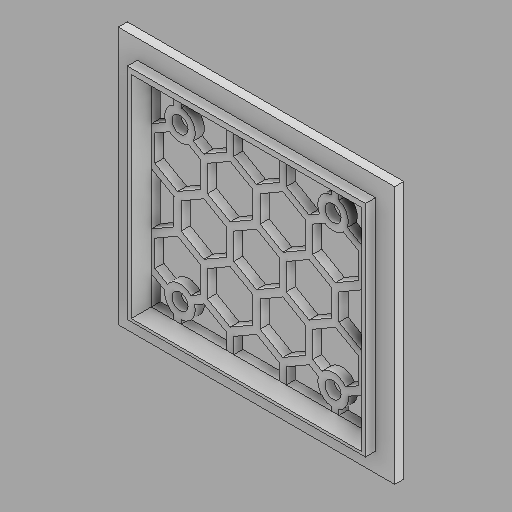
# Autodesk Inventor part: First_Stage_HexGrill
Saved by Autodesk Inventor 2025.2 (Build 292293000, 293)
## iProperties
Created: 2024-12-06
Part Number: First_Stage_HexGrill
Material: Generic
Document SubType Name: Modeling
Designer: Paul Linke
Density: 1 g/cm^3
Appearance: Default
Author: Paul Linke
Autodesk Inventor part; units mm, degrees
ref_plane "YZ Plane" through (0, 0, 0) normal (1, 0, 0) x (0, 1, 0)
ref_plane "XZ Plane" through (0, 0, 0) normal (0, 1, 0) x (-1, 0, 0)
ref_plane "Work Plane1" through (0, 0, 0) normal (0, 0, 1) x (1, 0, 0)
sketch "Sketch1" plane through (0, 0, 0) normal (0, 0, 1) x (1, 0, 0)
  line L0 (-29, 27) -> (-29, -27) projected
  line L1 (-25, -27) -> (-29, -27) projected
  line L2 (-25, 23) -> (-25, -27) projected
  line L3 (25, 23) -> (-25, 23) projected
  line L4 (25, -27) -> (25, 23) projected
  line L5 (29, -27) -> (25, -27) projected
  line L6 (29, -27) -> (29, 27) projected
  line L7 (-29, 27) -> (29, 27) projected
  line L8 (-29, 27) -> (-29, -27) projected
  line L9 (-25, -27) -> (-29, -27) projected
  line L10 (-25, 23) -> (-25, -27) projected
  line L11 (25, 23) -> (-25, 23) projected
  line L12 (25, -27) -> (25, 23) projected
  line L13 (29, -27) -> (25, -27) projected
  line L14 (29, -27) -> (29, 27) projected
  line L15 (-29, 27) -> (29, 27) projected
  line L16 (29, -27) -> (-29, -27)
  line L17 (-29, -27) -> (-29, 27)
  line L18 (-29, 27) -> (29, 27)
  line L19 (29, 27) -> (29, -27)
  line L20 (28.9, -27) -> (-28.9, -27)
  line L21 (-28.9, -27) -> (-28.9, 26.9)
  line L22 (-28.9, 26.9) -> (28.9, 26.9)
  line L23 (28.9, 26.9) -> (28.9, -27)
  line L24 (25, -27) -> (-25, -27)
  line L25 (-25, -27) -> (-25, 23)
  line L26 (-25, 23) -> (25, 23)
  line L27 (25, 23) -> (25, -23)
  line L28 (66.972, -23) -> (25, -23) projected
  line L29 (-25, -23) -> (-107.0316, -23) projected
  line L30 (-25, -23) -> (-25, -26.9)
  dimension "d0" = 0.1
  dimension "d1" = 0.1
  dimension "d2" = 0.1
  constraints: 26 end point, 6 parallel, 3 horizontal, 3 perpendicular, 2 point on line
  measures "d0" distance between parallel lines of L6 L23
  measures "d1" distance between parallel lines of L0 L21
  measures "d2" distance between parallel lines of L18 L22
extrude "Extrusion1" add sketch "Sketch1" along normal blind 1.9 contours L29 L2 L1 L21 | L21 L22 L23 L28 L4 L3 L2 L29 | L2 L3 L4 L16 | L23 L5 L4 L28
sketch "Sketch3" plane through (0, 0, 1.9) normal (0, 0, 1) x (1, 0, 0)
  line L0 (66.972, -23) -> (25, -23) projected
  line L1 (-25, -23) -> (-107.0316, -23) projected
  line L2 (25, 23) -> (25, -23) projected
  line L3 (-25, 23) -> (25, 23) projected
  line L4 (-25, -23) -> (-25, 23) projected
  line L5 (24.9, -23) -> (-24.9, -23)
  line L6 (-24.9, -23) -> (-24.9, 22.9)
  line L7 (-24.9, 22.9) -> (24.9, 22.9)
  line L8 (24.9, 22.9) -> (24.9, -23)
  point P0 (0, 0)
  dimension "d18" = 0.1
  dimension "d19" = 0.1
  dimension "d20" = 0.1
  constraints: 8 end point, 2 parallel, 1 collinear, 1 horizontal, 1 perpendicular
  measures "d18" distance between parallel lines of L2 L8
  measures "d19" distance between parallel lines of L3 L7
  measures "d20" distance between parallel lines of L4 L6
extrude "Extrusion3" add sketch "Sketch3" along normal blind 2.1
sketch "Sketch4" plane through (0, 0, 4) normal (0, 0, 1) x (1, 0, 0)
  line L0 (-24.9, -23) -> (24.9, -23) projected
  line L1 (24.9, 22.9) -> (-24.9, 22.9) projected
  line L2 (-24.9, 22.9) -> (-24.9, -23) projected
  line L3 (-24.9, -23) -> (24.9, -23) projected
  line L4 (24.9, -23) -> (24.9, 22.9) projected
  line L5 (24.9, -23) -> (-24.9, 22.9) construction
  line L6 (24.9, 22.9) -> (-24.9, -23) construction
  line L7 (22, -20.3271) -> (-22, -20.3271)
  line L8 (-22, -20.3271) -> (-22, 19.6729)
  line L9 (-22, 19.6729) -> (22, 19.6729)
  line L10 (22, 19.6729) -> (22, -20.3271)
  point P0 (0, 0)
  dimension "d23" = 44
  dimension "d24" = 40
  constraints: 12 end point, 2 parallel, 2 point on line, 1 horizontal, 1 perpendicular
  measures "d23" distance between parallel lines of L8 L10
  measures "d24" distance between parallel lines of L9 L7
extrude "Extrusion4" cut sketch "Sketch4" against normal blind 2.1 contours L7 L8 L9 L10
chamfer "Chamfer1" distance 2.1 angle 45 4 edges at (0, -20.3271, 4) (-22, -0.3271, 4) (0, 19.6729, 4) (22, -0.3271, 4)
sketch "Sketch5" plane through (0, 0, 1.9) normal (0, 0, 1) x (1, 0, 0)
  line L0 (-43.092, -0.7164) -> (45.2522, -0.7164) construction
  line L1 (-44, 4.7684) -> (-39.25, 2.026)
  line L2 (-39.25, 2.026) -> (-39.25, -3.4588)
  line L3 (-39.25, -3.4588) -> (-44, -6.2012)
  line L4 (-44, -6.2012) -> (-48.75, -3.4588)
  line L5 (-48.75, -3.4588) -> (-48.75, 2.026)
  line L6 (-48.75, 2.026) -> (-44, 4.7684)
  line L7 (-44, 4.7684) -> (-44, -6.2012) construction
  circle A0 centre (-16, 15.6729) radius 1.7
  circle A1 centre (16, 15.6729) radius 1.7
  circle A2 centre (-16, -16.3271) radius 1.7
  circle A3 centre (16, -16.3271) radius 1.7
  line L8 (-24.1, -22.4271) -> (-22, -20.3271) projected
  line L9 (-16, 15.6729) -> (-22, 15.6729) construction
  line L10 (-22, -20.3271) -> (-22, 19.6729) projected
  line L11 (16, 15.6729) -> (22, 15.6729) construction
  line L12 (22, 19.6729) -> (22, -20.3271) projected
  line L13 (-16, 15.6729) -> (-16, 19.6729) construction
  line L14 (-22, 19.6729) -> (22, 19.6729) projected
  line L15 (-16, -16.3271) -> (-16, -20.3271) construction
  line L16 (22, -20.3271) -> (-22, -20.3271) construction
  line L17 (-44, -0.7164) -> (-41.625, 3.3972) construction
  line L18 (-28.25, 2.026) -> (-28.25, -3.4588)
  line L19 (-28.25, -3.4588) -> (-33, -6.2012)
  line L20 (-33, 4.7684) -> (-28.25, 2.026)
  line L21 (-33, -6.2012) -> (-37.75, -3.4588)
  line L22 (-37.75, -3.4588) -> (-37.75, 2.026)
  line L23 (-37.75, 2.026) -> (-33, 4.7684)
  line L24 (-17.25, 2.026) -> (-17.25, -3.4588)
  line L25 (-17.25, -3.4588) -> (-22, -6.2012)
  line L26 (-22, 4.7684) -> (-17.25, 2.026)
  line L27 (-22, -6.2012) -> (-26.75, -3.4588)
  line L28 (-26.75, -3.4588) -> (-26.75, 2.026)
  line L29 (-26.75, 2.026) -> (-22, 4.7684)
  line L30 (-6.25, 2.026) -> (-6.25, -3.4588)
  line L31 (-6.25, -3.4588) -> (-11, -6.2012)
  line L32 (-11, 4.7684) -> (-6.25, 2.026)
  line L33 (-11, -6.2012) -> (-15.75, -3.4588)
  line L34 (-15.75, -3.4588) -> (-15.75, 2.026)
  line L35 (-15.75, 2.026) -> (-11, 4.7684)
  line L36 (4.75, 2.026) -> (4.75, -3.4588)
  line L37 (4.75, -3.4588) -> (0, -6.2012)
  line L38 (0, 4.7684) -> (4.75, 2.026)
  line L39 (0, -6.2012) -> (-4.75, -3.4588)
  line L40 (-4.75, -3.4588) -> (-4.75, 2.026)
  line L41 (-4.75, 2.026) -> (0, 4.7684)
  line L42 (15.75, 2.026) -> (15.75, -3.4588)
  line L43 (15.75, -3.4588) -> (11, -6.2012)
  line L44 (11, 4.7684) -> (15.75, 2.026)
  line L45 (11, -6.2012) -> (6.25, -3.4588)
  line L46 (6.25, -3.4588) -> (6.25, 2.026)
  line L47 (6.25, 2.026) -> (11, 4.7684)
  line L48 (26.75, 2.026) -> (26.75, -3.4588)
  line L49 (26.75, -3.4588) -> (22, -6.2012)
  line L50 (22, 4.7684) -> (26.75, 2.026)
  line L51 (22, -6.2012) -> (17.25, -3.4588)
  line L52 (17.25, -3.4588) -> (17.25, 2.026)
  line L53 (17.25, 2.026) -> (22, 4.7684)
  line L54 (37.75, 2.026) -> (37.75, -3.4588)
  line L55 (37.75, -3.4588) -> (33, -6.2012)
  line L56 (33, 4.7684) -> (37.75, 2.026)
  line L57 (33, -6.2012) -> (28.25, -3.4588)
  line L58 (28.25, -3.4588) -> (28.25, 2.026)
  line L59 (28.25, 2.026) -> (33, 4.7684)
  line L60 (48.75, 2.026) -> (48.75, -3.4588)
  line L61 (48.75, -3.4588) -> (44, -6.2012)
  line L62 (44, 4.7684) -> (48.75, 2.026)
  line L63 (44, -6.2012) -> (39.25, -3.4588)
  line L64 (39.25, -3.4588) -> (39.25, 2.026)
  line L65 (39.25, 2.026) -> (44, 4.7684)
  line L66 (59.75, 2.026) -> (59.75, -3.4588)
  line L67 (59.75, -3.4588) -> (55, -6.2012)
  line L68 (55, 4.7684) -> (59.75, 2.026)
  line L69 (55, -6.2012) -> (50.25, -3.4588)
  line L70 (50.25, -3.4588) -> (50.25, 2.026)
  line L71 (50.25, 2.026) -> (55, 4.7684)
  line L72 (-11.75, 6.0675) -> (-16.5, 3.3251)
  line L73 (-11.75, 11.5523) -> (-11.75, 6.0675)
  line L74 (-16.5, 14.2947) -> (-11.75, 11.5523)
  line L75 (-5.5, 3.3251) -> (-10.25, 6.0675)
  line L76 (-10.25, 11.5523) -> (-5.5, 14.2947)
  line L77 (-0.75, 6.0675) -> (-5.5, 3.3251)
  line L78 (-0.75, 11.5523) -> (-0.75, 6.0675)
  line L79 (-5.5, 14.2947) -> (-0.75, 11.5523)
  line L80 (-37.592, 8.8099) -> (50.7522, 8.8099) construction
  line L81 (-10.25, 6.0675) -> (-10.25, 11.5523)
  line L82 (-16.5, 3.3251) -> (-21.25, 6.0675)
  line L83 (-21.25, 6.0675) -> (-21.25, 11.5523)
  line L84 (-21.25, 11.5523) -> (-16.5, 14.2947)
  line L85 (0.75, 6.0675) -> (0.75, 11.5523)
  line L86 (0.75, 11.5523) -> (5.5, 14.2947)
  line L87 (5.5, 3.3251) -> (0.75, 6.0675)
  line L88 (10.25, 6.0675) -> (5.5, 3.3251)
  line L89 (5.5, 14.2947) -> (10.25, 11.5523)
  line L90 (11.75, 6.0675) -> (11.75, 11.5523)
  line L91 (16.5, 3.3251) -> (11.75, 6.0675)
  line L92 (11.75, 11.5523) -> (16.5, 14.2947)
  line L93 (10.25, 11.5523) -> (10.25, 6.0675)
  line L94 (32.25, 6.0675) -> (27.5, 3.3251)
  line L95 (32.25, 11.5523) -> (32.25, 6.0675)
  line L96 (33.75, 6.0675) -> (33.75, 11.5523)
  line L97 (38.5, 3.3251) -> (33.75, 6.0675)
  line L98 (33.75, 11.5523) -> (38.5, 14.2947)
  line L99 (43.25, 6.0675) -> (38.5, 3.3251)
  line L100 (43.25, 11.5523) -> (43.25, 6.0675)
  line L101 (38.5, 14.2947) -> (43.25, 11.5523)
  line L102 (27.5, 14.2947) -> (32.25, 11.5523)
  line L103 (27.5, 3.3251) -> (22.75, 6.0675)
  line L104 (22.75, 11.5523) -> (27.5, 14.2947)
  line L105 (22.75, 6.0675) -> (22.75, 11.5523)
  line L106 (16.5, 14.2947) -> (21.25, 11.5523)
  line L107 (21.25, 6.0675) -> (16.5, 3.3251)
  line L108 (21.25, 11.5523) -> (21.25, 6.0675)
  line L109 (-38.5, 14.2947) -> (-33.75, 11.5523)
  line L110 (-33.75, 11.5523) -> (-33.75, 6.0675)
  line L111 (-33.75, 6.0675) -> (-38.5, 3.3251)
  line L112 (-38.5, 3.3251) -> (-43.25, 6.0675)
  line L113 (-43.25, 6.0675) -> (-43.25, 11.5523)
  line L114 (-43.25, 11.5523) -> (-38.5, 14.2947)
  line L115 (-38.5, 14.2947) -> (-38.5, 3.3251) construction
  line L116 (-22.75, 11.5523) -> (-22.75, 6.0675)
  line L117 (-22.75, 6.0675) -> (-27.5, 3.3251)
  line L118 (-27.5, 14.2947) -> (-22.75, 11.5523)
  line L119 (-27.5, 3.3251) -> (-32.25, 6.0675)
  line L120 (-32.25, 11.5523) -> (-27.5, 14.2947)
  line L121 (-32.25, 6.0675) -> (-32.25, 11.5523)
  line L122 (44.75, 6.0675) -> (44.75, 11.5523)
  line L123 (44.75, 11.5523) -> (49.5, 14.2947)
  line L124 (49.5, 3.3251) -> (44.75, 6.0675)
  line L125 (54.25, 6.0675) -> (49.5, 3.3251)
  line L126 (49.5, 14.2947) -> (54.25, 11.5523)
  line L127 (54.25, 11.5523) -> (54.25, 6.0675)
  line L128 (55.75, 6.0675) -> (55.75, 11.5523)
  line L129 (60.5, 3.3251) -> (55.75, 6.0675)
  line L130 (65.25, 6.0675) -> (60.5, 3.3251)
  line L131 (65.25, 11.5523) -> (65.25, 6.0675)
  line L132 (60.5, 14.2947) -> (65.25, 11.5523)
  line L133 (55.75, 11.5523) -> (60.5, 14.2947)
  line L134 (-6.25, 15.5937) -> (-11, 12.8513)
  line L135 (-6.25, 21.0786) -> (-6.25, 15.5937)
  line L136 (-11, 23.821) -> (-6.25, 21.0786)
  line L137 (0, 12.8513) -> (-4.75, 15.5937)
  line L138 (-4.75, 21.0786) -> (0, 23.821)
  line L139 (4.75, 15.5937) -> (0, 12.8513)
  line L140 (4.75, 21.0786) -> (4.75, 15.5937)
  line L141 (0, 23.821) -> (4.75, 21.0786)
  line L142 (-32.092, 18.3362) -> (56.2522, 18.3362) construction
  line L143 (-4.75, 15.5937) -> (-4.75, 21.0786)
  line L144 (-11, 12.8513) -> (-15.75, 15.5937)
  line L145 (-15.75, 15.5937) -> (-15.75, 21.0786)
  line L146 (-15.75, 21.0786) -> (-11, 23.821)
  line L147 (6.25, 15.5937) -> (6.25, 21.0786)
  line L148 (6.25, 21.0786) -> (11, 23.821)
  line L149 (11, 12.8513) -> (6.25, 15.5937)
  line L150 (15.75, 15.5937) -> (11, 12.8513)
  line L151 (11, 23.821) -> (15.75, 21.0786)
  line L152 (17.25, 15.5937) -> (17.25, 21.0786)
  line L153 (22, 12.8513) -> (17.25, 15.5937)
  line L154 (17.25, 21.0786) -> (22, 23.821)
  line L155 (15.75, 21.0786) -> (15.75, 15.5937)
  line L156 (37.75, 15.5937) -> (33, 12.8513)
  line L157 (37.75, 21.0786) -> (37.75, 15.5937)
  line L158 (39.25, 15.5937) -> (39.25, 21.0786)
  line L159 (44, 12.8513) -> (39.25, 15.5937)
  line L160 (39.25, 21.0786) -> (44, 23.821)
  line L161 (48.75, 15.5937) -> (44, 12.8513)
  line L162 (48.75, 21.0786) -> (48.75, 15.5937)
  line L163 (44, 23.821) -> (48.75, 21.0786)
  line L164 (33, 23.821) -> (37.75, 21.0786)
  line L165 (33, 12.8513) -> (28.25, 15.5937)
  line L166 (28.25, 21.0786) -> (33, 23.821)
  line L167 (28.25, 15.5937) -> (28.25, 21.0786)
  line L168 (22, 23.821) -> (26.75, 21.0786)
  line L169 (26.75, 15.5937) -> (22, 12.8513)
  line L170 (26.75, 21.0786) -> (26.75, 15.5937)
  line L171 (-33, 23.821) -> (-28.25, 21.0786)
  line L172 (-28.25, 21.0786) -> (-28.25, 15.5937)
  line L173 (-28.25, 15.5937) -> (-33, 12.8513)
  line L174 (-33, 12.8513) -> (-37.75, 15.5937)
  line L175 (-37.75, 15.5937) -> (-37.75, 21.0786)
  line L176 (-37.75, 21.0786) -> (-33, 23.821)
  line L177 (-33, 23.821) -> (-33, 12.8513) construction
  line L178 (-17.25, 21.0786) -> (-17.25, 15.5937)
  line L179 (-17.25, 15.5937) -> (-22, 12.8513)
  line L180 (-22, 23.821) -> (-17.25, 21.0786)
  line L181 (-22, 12.8513) -> (-26.75, 15.5937)
  line L182 (-26.75, 21.0786) -> (-22, 23.821)
  line L183 (-26.75, 15.5937) -> (-26.75, 21.0786)
  line L184 (50.25, 15.5937) -> (50.25, 21.0786)
  line L185 (50.25, 21.0786) -> (55, 23.821)
  line L186 (55, 12.8513) -> (50.25, 15.5937)
  line L187 (59.75, 15.5937) -> (55, 12.8513)
  line L188 (55, 23.821) -> (59.75, 21.0786)
  line L189 (59.75, 21.0786) -> (59.75, 15.5937)
  line L190 (61.25, 15.5937) -> (61.25, 21.0786)
  line L191 (66, 12.8513) -> (61.25, 15.5937)
  line L192 (70.75, 15.5937) -> (66, 12.8513)
  line L193 (70.75, 21.0786) -> (70.75, 15.5937)
  line L194 (66, 23.821) -> (70.75, 21.0786)
  line L195 (61.25, 21.0786) -> (66, 23.821)
  line L196 (-0.75, 25.12) -> (-5.5, 22.3776)
  line L197 (-0.75, 30.6049) -> (-0.75, 25.12)
  line L198 (-5.5, 33.3473) -> (-0.75, 30.6049)
  line L199 (5.5, 22.3776) -> (0.75, 25.12)
  line L200 (0.75, 30.6049) -> (5.5, 33.3473)
  line L201 (10.25, 25.12) -> (5.5, 22.3776)
  line L202 (10.25, 30.6049) -> (10.25, 25.12)
  line L203 (5.5, 33.3473) -> (10.25, 30.6049)
  line L204 (-26.592, 27.8624) -> (61.7522, 27.8624) construction
  line L205 (0.75, 25.12) -> (0.75, 30.6049)
  line L206 (-5.5, 22.3776) -> (-10.25, 25.12)
  line L207 (-10.25, 25.12) -> (-10.25, 30.6049)
  line L208 (-10.25, 30.6049) -> (-5.5, 33.3473)
  line L209 (11.75, 25.12) -> (11.75, 30.6049)
  line L210 (11.75, 30.6049) -> (16.5, 33.3473)
  line L211 (16.5, 22.3776) -> (11.75, 25.12)
  line L212 (21.25, 25.12) -> (16.5, 22.3776)
  line L213 (16.5, 33.3473) -> (21.25, 30.6049)
  line L214 (22.75, 25.12) -> (22.75, 30.6049)
  line L215 (27.5, 22.3776) -> (22.75, 25.12)
  line L216 (22.75, 30.6049) -> (27.5, 33.3473)
  line L217 (21.25, 30.6049) -> (21.25, 25.12)
  line L218 (43.25, 25.12) -> (38.5, 22.3776)
  line L219 (43.25, 30.6049) -> (43.25, 25.12)
  line L220 (44.75, 25.12) -> (44.75, 30.6049)
  line L221 (49.5, 22.3776) -> (44.75, 25.12)
  line L222 (44.75, 30.6049) -> (49.5, 33.3473)
  line L223 (54.25, 25.12) -> (49.5, 22.3776)
  line L224 (54.25, 30.6049) -> (54.25, 25.12)
  line L225 (49.5, 33.3473) -> (54.25, 30.6049)
  line L226 (38.5, 33.3473) -> (43.25, 30.6049)
  line L227 (38.5, 22.3776) -> (33.75, 25.12)
  line L228 (33.75, 30.6049) -> (38.5, 33.3473)
  line L229 (33.75, 25.12) -> (33.75, 30.6049)
  line L230 (27.5, 33.3473) -> (32.25, 30.6049)
  line L231 (32.25, 25.12) -> (27.5, 22.3776)
  line L232 (32.25, 30.6049) -> (32.25, 25.12)
  line L233 (-27.5, 33.3473) -> (-22.75, 30.6049)
  line L234 (-22.75, 30.6049) -> (-22.75, 25.12)
  line L235 (-22.75, 25.12) -> (-27.5, 22.3776)
  line L236 (-27.5, 22.3776) -> (-32.25, 25.12)
  line L237 (-32.25, 25.12) -> (-32.25, 30.6049)
  line L238 (-32.25, 30.6049) -> (-27.5, 33.3473)
  line L239 (-27.5, 33.3473) -> (-27.5, 22.3776) construction
  line L240 (-11.75, 30.6049) -> (-11.75, 25.12)
  line L241 (-11.75, 25.12) -> (-16.5, 22.3776)
  line L242 (-16.5, 33.3473) -> (-11.75, 30.6049)
  line L243 (-16.5, 22.3776) -> (-21.25, 25.12)
  line L244 (-21.25, 30.6049) -> (-16.5, 33.3473)
  line L245 (-21.25, 25.12) -> (-21.25, 30.6049)
  line L246 (55.75, 25.12) -> (55.75, 30.6049)
  line L247 (55.75, 30.6049) -> (60.5, 33.3473)
  line L248 (60.5, 22.3776) -> (55.75, 25.12)
  line L249 (65.25, 25.12) -> (60.5, 22.3776)
  line L250 (60.5, 33.3473) -> (65.25, 30.6049)
  line L251 (65.25, 30.6049) -> (65.25, 25.12)
  line L252 (66.75, 25.12) -> (66.75, 30.6049)
  line L253 (71.5, 22.3776) -> (66.75, 25.12)
  line L254 (76.25, 25.12) -> (71.5, 22.3776)
  line L255 (76.25, 30.6049) -> (76.25, 25.12)
  line L256 (71.5, 33.3473) -> (76.25, 30.6049)
  line L257 (66.75, 30.6049) -> (71.5, 33.3473)
  line L258 (-48.592, -10.2427) -> (39.7522, -10.2427) construction
  line L259 (32.25, -7.5003) -> (32.25, -12.9851)
  line L260 (32.25, -12.9851) -> (27.5, -15.7275)
  line L261 (27.5, -4.7579) -> (32.25, -7.5003)
  line L262 (27.5, -15.7275) -> (22.75, -12.9851)
  line L263 (22.75, -12.9851) -> (22.75, -7.5003)
  line L264 (22.75, -7.5003) -> (27.5, -4.7579)
  line L265 (26.75, -3.4588) -> (22, -6.2012)
  line L266 (33, -6.2012) -> (28.25, -3.4588)
  line L267 (15.75, -3.4588) -> (11, -6.2012)
  line L268 (22, -6.2012) -> (17.25, -3.4588)
  line L269 (11.75, -7.5003) -> (16.5, -4.7579)
  line L270 (16.5, -4.7579) -> (21.25, -7.5003)
  line L271 (21.25, -7.5003) -> (21.25, -12.9851)
  line L272 (11.75, -12.9851) -> (11.75, -7.5003)
  line L273 (16.5, -15.7275) -> (11.75, -12.9851)
  line L274 (21.25, -12.9851) -> (16.5, -15.7275)
  line L275 (-0.75, -7.5003) -> (-0.75, -12.9851)
  line L276 (-0.75, -12.9851) -> (-5.5, -15.7275)
  line L277 (10.25, -7.5003) -> (10.25, -12.9851)
  line L278 (5.5, -4.7579) -> (10.25, -7.5003)
  line L279 (0.75, -7.5003) -> (5.5, -4.7579)
  line L280 (0.75, -12.9851) -> (0.75, -7.5003)
  line L281 (5.5, -15.7275) -> (0.75, -12.9851)
  line L282 (10.25, -12.9851) -> (5.5, -15.7275)
  line L283 (-5.5, -4.7579) -> (-0.75, -7.5003)
  line L284 (11, -6.2012) -> (6.25, -3.4588)
  line L285 (4.75, -3.4588) -> (0, -6.2012)
  line L286 (0, -6.2012) -> (-4.75, -3.4588)
  line L287 (-11, -6.2012) -> (-15.75, -3.4588)
  line L288 (-16.5, -4.7579) -> (-11.75, -7.5003)
  line L289 (-17.25, -3.4588) -> (-22, -6.2012)
  line L290 (-6.25, -3.4588) -> (-11, -6.2012)
  line L291 (-21.25, -7.5003) -> (-16.5, -4.7579)
  line L292 (-10.25, -7.5003) -> (-5.5, -4.7579)
  line L293 (-11.75, -7.5003) -> (-11.75, -12.9851)
  line L294 (-10.25, -12.9851) -> (-10.25, -7.5003)
  line L295 (-21.25, -12.9851) -> (-21.25, -7.5003)
  line L296 (-5.5, -15.7275) -> (-10.25, -12.9851)
  line L297 (-11.75, -12.9851) -> (-16.5, -15.7275)
  line L298 (-16.5, -15.7275) -> (-21.25, -12.9851)
  line L299 (-33.75, -7.5003) -> (-33.75, -12.9851)
  line L300 (-33.75, -12.9851) -> (-38.5, -15.7275)
  line L301 (-22.75, -7.5003) -> (-22.75, -12.9851)
  line L302 (-22.75, -12.9851) -> (-27.5, -15.7275)
  line L303 (-27.5, -4.7579) -> (-22.75, -7.5003)
  line L304 (-27.5, -15.7275) -> (-32.25, -12.9851)
  line L305 (-32.25, -12.9851) -> (-32.25, -7.5003)
  line L306 (-32.25, -7.5003) -> (-27.5, -4.7579)
  line L307 (-22, -6.2012) -> (-26.75, -3.4588)
  line L308 (-33, -6.2012) -> (-37.75, -3.4588)
  line L309 (-28.25, -3.4588) -> (-33, -6.2012)
  line L310 (43.25, -7.5003) -> (43.25, -12.9851)
  line L311 (43.25, -12.9851) -> (38.5, -15.7275)
  line L312 (38.5, -4.7579) -> (43.25, -7.5003)
  line L313 (38.5, -15.7275) -> (33.75, -12.9851)
  line L314 (33.75, -12.9851) -> (33.75, -7.5003)
  line L315 (33.75, -7.5003) -> (38.5, -4.7579)
  line L316 (37.75, -3.4588) -> (33, -6.2012)
  line L317 (44, -6.2012) -> (39.25, -3.4588)
  line L318 (48.75, -3.4588) -> (44, -6.2012)
  line L319 (44.75, -7.5003) -> (49.5, -4.7579)
  line L320 (44.75, -12.9851) -> (44.75, -7.5003)
  line L321 (49.5, -15.7275) -> (44.75, -12.9851)
  line L322 (49.5, -4.7579) -> (54.25, -7.5003)
  line L323 (55, -6.2012) -> (50.25, -3.4588)
  line L324 (59.75, -3.4588) -> (55, -6.2012)
  line L325 (54.25, -7.5003) -> (54.25, -12.9851)
  line L326 (54.25, -12.9851) -> (49.5, -15.7275)
  line L327 (-38.5, -4.7579) -> (-33.75, -7.5003)
  line L328 (-43.25, -7.5003) -> (-38.5, -4.7579)
  line L329 (-44, -6.2012) -> (-48.75, -3.4588)
  line L330 (-39.25, -3.4588) -> (-44, -6.2012)
  line L331 (-49.5, -4.7579) -> (-44.75, -7.5003)
  line L332 (-44.75, -7.5003) -> (-44.75, -12.9851)
  line L333 (-44.75, -12.9851) -> (-49.5, -15.7275)
  line L334 (-49.5, -15.7275) -> (-54.25, -12.9851)
  line L335 (-54.25, -12.9851) -> (-54.25, -7.5003)
  line L336 (-54.25, -7.5003) -> (-49.5, -4.7579)
  line L337 (-49.5, -4.7579) -> (-49.5, -15.7275) construction
  line L338 (-49.5, -10.2427) -> (-47.125, -6.1291) construction
  line L339 (-38.5, -15.7275) -> (-43.25, -12.9851)
  line L340 (-43.25, -12.9851) -> (-43.25, -7.5003)
  line L341 (-54.092, -19.769) -> (34.2522, -19.769) construction
  line L342 (26.75, -17.0265) -> (26.75, -22.5114)
  line L343 (26.75, -22.5114) -> (22, -25.2538)
  line L344 (22, -14.2841) -> (26.75, -17.0265)
  line L345 (22, -25.2538) -> (17.25, -22.5114)
  line L346 (17.25, -22.5114) -> (17.25, -17.0265)
  line L347 (17.25, -17.0265) -> (22, -14.2841)
  line L348 (21.25, -12.9851) -> (16.5, -15.7275)
  line L349 (27.5, -15.7275) -> (22.75, -12.9851)
  line L350 (10.25, -12.9851) -> (5.5, -15.7275)
  line L351 (16.5, -15.7275) -> (11.75, -12.9851)
  line L352 (6.25, -17.0265) -> (11, -14.2841)
  line L353 (11, -14.2841) -> (15.75, -17.0265)
  line L354 (15.75, -17.0265) -> (15.75, -22.5114)
  line L355 (6.25, -22.5114) -> (6.25, -17.0265)
  line L356 (11, -25.2538) -> (6.25, -22.5114)
  line L357 (15.75, -22.5114) -> (11, -25.2538)
  line L358 (-6.25, -17.0265) -> (-6.25, -22.5114)
  line L359 (-6.25, -22.5114) -> (-11, -25.2538)
  line L360 (4.75, -17.0265) -> (4.75, -22.5114)
  line L361 (0, -14.2841) -> (4.75, -17.0265)
  line L362 (-4.75, -17.0265) -> (0, -14.2841)
  line L363 (-4.75, -22.5114) -> (-4.75, -17.0265)
  line L364 (0, -25.2538) -> (-4.75, -22.5114)
  line L365 (4.75, -22.5114) -> (0, -25.2538)
  line L366 (-11, -14.2841) -> (-6.25, -17.0265)
  line L367 (5.5, -15.7275) -> (0.75, -12.9851)
  line L368 (-0.75, -12.9851) -> (-5.5, -15.7275)
  line L369 (-5.5, -15.7275) -> (-10.25, -12.9851)
  line L370 (-16.5, -15.7275) -> (-21.25, -12.9851)
  line L371 (-22, -14.2841) -> (-17.25, -17.0265)
  line L372 (-22.75, -12.9851) -> (-27.5, -15.7275)
  line L373 (-11.75, -12.9851) -> (-16.5, -15.7275)
  line L374 (-26.75, -17.0265) -> (-22, -14.2841)
  line L375 (-15.75, -17.0265) -> (-11, -14.2841)
  line L376 (-17.25, -17.0265) -> (-17.25, -22.5114)
  line L377 (-15.75, -22.5114) -> (-15.75, -17.0265)
  line L378 (-26.75, -22.5114) -> (-26.75, -17.0265)
  line L379 (-11, -25.2538) -> (-15.75, -22.5114)
  line L380 (-17.25, -22.5114) -> (-22, -25.2538)
  line L381 (-22, -25.2538) -> (-26.75, -22.5114)
  line L382 (-39.25, -17.0265) -> (-39.25, -22.5114)
  line L383 (-39.25, -22.5114) -> (-44, -25.2538)
  line L384 (-28.25, -17.0265) -> (-28.25, -22.5114)
  line L385 (-28.25, -22.5114) -> (-33, -25.2538)
  line L386 (-33, -14.2841) -> (-28.25, -17.0265)
  line L387 (-33, -25.2538) -> (-37.75, -22.5114)
  line L388 (-37.75, -22.5114) -> (-37.75, -17.0265)
  line L389 (-37.75, -17.0265) -> (-33, -14.2841)
  line L390 (-27.5, -15.7275) -> (-32.25, -12.9851)
  line L391 (-38.5, -15.7275) -> (-43.25, -12.9851)
  line L392 (-33.75, -12.9851) -> (-38.5, -15.7275)
  line L393 (37.75, -17.0265) -> (37.75, -22.5114)
  line L394 (37.75, -22.5114) -> (33, -25.2538)
  line L395 (33, -14.2841) -> (37.75, -17.0265)
  line L396 (33, -25.2538) -> (28.25, -22.5114)
  line L397 (28.25, -22.5114) -> (28.25, -17.0265)
  line L398 (28.25, -17.0265) -> (33, -14.2841)
  line L399 (32.25, -12.9851) -> (27.5, -15.7275)
  line L400 (38.5, -15.7275) -> (33.75, -12.9851)
  line L401 (43.25, -12.9851) -> (38.5, -15.7275)
  line L402 (39.25, -17.0265) -> (44, -14.2841)
  line L403 (39.25, -22.5114) -> (39.25, -17.0265)
  line L404 (44, -25.2538) -> (39.25, -22.5114)
  line L405 (44, -14.2841) -> (48.75, -17.0265)
  line L406 (49.5, -15.7275) -> (44.75, -12.9851)
  line L407 (54.25, -12.9851) -> (49.5, -15.7275)
  line L408 (48.75, -17.0265) -> (48.75, -22.5114)
  line L409 (48.75, -22.5114) -> (44, -25.2538)
  line L410 (-44, -14.2841) -> (-39.25, -17.0265)
  line L411 (-48.75, -17.0265) -> (-44, -14.2841)
  line L412 (-49.5, -15.7275) -> (-54.25, -12.9851)
  line L413 (-44.75, -12.9851) -> (-49.5, -15.7275)
  line L414 (-55, -14.2841) -> (-50.25, -17.0265)
  line L415 (-50.25, -17.0265) -> (-50.25, -22.5114)
  line L416 (-50.25, -22.5114) -> (-55, -25.2538)
  line L417 (-55, -25.2538) -> (-59.75, -22.5114)
  line L418 (-59.75, -22.5114) -> (-59.75, -17.0265)
  line L419 (-59.75, -17.0265) -> (-55, -14.2841)
  line L420 (-55, -14.2841) -> (-55, -25.2538) construction
  line L421 (-55, -19.769) -> (-52.625, -15.6553) construction
  line L422 (-44, -25.2538) -> (-48.75, -22.5114)
  line L423 (-48.75, -22.5114) -> (-48.75, -17.0265)
  line L424 (-59.592, -29.2952) -> (28.7522, -29.2952) construction
  line L425 (21.25, -26.5528) -> (21.25, -32.0377)
  line L426 (21.25, -32.0377) -> (16.5, -34.7801)
  line L427 (16.5, -23.8104) -> (21.25, -26.5528)
  line L428 (16.5, -34.7801) -> (11.75, -32.0377)
  line L429 (11.75, -32.0377) -> (11.75, -26.5528)
  line L430 (11.75, -26.5528) -> (16.5, -23.8104)
  line L431 (15.75, -22.5114) -> (11, -25.2538)
  line L432 (22, -25.2538) -> (17.25, -22.5114)
  line L433 (4.75, -22.5114) -> (0, -25.2538)
  line L434 (11, -25.2538) -> (6.25, -22.5114)
  line L435 (0.75, -26.5528) -> (5.5, -23.8104)
  line L436 (5.5, -23.8104) -> (10.25, -26.5528)
  line L437 (10.25, -26.5528) -> (10.25, -32.0377)
  line L438 (0.75, -32.0377) -> (0.75, -26.5528)
  line L439 (5.5, -34.7801) -> (0.75, -32.0377)
  line L440 (10.25, -32.0377) -> (5.5, -34.7801)
  line L441 (-11.75, -26.5528) -> (-11.75, -32.0377)
  line L442 (-11.75, -32.0377) -> (-16.5, -34.7801)
  line L443 (-0.75, -26.5528) -> (-0.75, -32.0377)
  line L444 (-5.5, -23.8104) -> (-0.75, -26.5528)
  line L445 (-10.25, -26.5528) -> (-5.5, -23.8104)
  line L446 (-10.25, -32.0377) -> (-10.25, -26.5528)
  line L447 (-5.5, -34.7801) -> (-10.25, -32.0377)
  line L448 (-0.75, -32.0377) -> (-5.5, -34.7801)
  line L449 (-16.5, -23.8104) -> (-11.75, -26.5528)
  line L450 (0, -25.2538) -> (-4.75, -22.5114)
  line L451 (-6.25, -22.5114) -> (-11, -25.2538)
  line L452 (-11, -25.2538) -> (-15.75, -22.5114)
  line L453 (-22, -25.2538) -> (-26.75, -22.5114)
  line L454 (-27.5, -23.8104) -> (-22.75, -26.5528)
  line L455 (-28.25, -22.5114) -> (-33, -25.2538)
  line L456 (-17.25, -22.5114) -> (-22, -25.2538)
  line L457 (-32.25, -26.5528) -> (-27.5, -23.8104)
  line L458 (-21.25, -26.5528) -> (-16.5, -23.8104)
  line L459 (-22.75, -26.5528) -> (-22.75, -32.0377)
  line L460 (-21.25, -32.0377) -> (-21.25, -26.5528)
  line L461 (-32.25, -32.0377) -> (-32.25, -26.5528)
  line L462 (-16.5, -34.7801) -> (-21.25, -32.0377)
  line L463 (-22.75, -32.0377) -> (-27.5, -34.7801)
  line L464 (-27.5, -34.7801) -> (-32.25, -32.0377)
  line L465 (-44.75, -26.5528) -> (-44.75, -32.0377)
  line L466 (-44.75, -32.0377) -> (-49.5, -34.7801)
  line L467 (-33.75, -26.5528) -> (-33.75, -32.0377)
  line L468 (-33.75, -32.0377) -> (-38.5, -34.7801)
  line L469 (-38.5, -23.8104) -> (-33.75, -26.5528)
  line L470 (-38.5, -34.7801) -> (-43.25, -32.0377)
  line L471 (-43.25, -32.0377) -> (-43.25, -26.5528)
  line L472 (-43.25, -26.5528) -> (-38.5, -23.8104)
  line L473 (-33, -25.2538) -> (-37.75, -22.5114)
  line L474 (-44, -25.2538) -> (-48.75, -22.5114)
  line L475 (-39.25, -22.5114) -> (-44, -25.2538)
  line L476 (32.25, -26.5528) -> (32.25, -32.0377)
  line L477 (32.25, -32.0377) -> (27.5, -34.7801)
  line L478 (27.5, -23.8104) -> (32.25, -26.5528)
  line L479 (27.5, -34.7801) -> (22.75, -32.0377)
  line L480 (22.75, -32.0377) -> (22.75, -26.5528)
  line L481 (22.75, -26.5528) -> (27.5, -23.8104)
  line L482 (26.75, -22.5114) -> (22, -25.2538)
  line L483 (33, -25.2538) -> (28.25, -22.5114)
  line L484 (37.75, -22.5114) -> (33, -25.2538)
  line L485 (33.75, -26.5528) -> (38.5, -23.8104)
  line L486 (33.75, -32.0377) -> (33.75, -26.5528)
  line L487 (38.5, -34.7801) -> (33.75, -32.0377)
  line L488 (38.5, -23.8104) -> (43.25, -26.5528)
  line L489 (44, -25.2538) -> (39.25, -22.5114)
  line L490 (48.75, -22.5114) -> (44, -25.2538)
  line L491 (43.25, -26.5528) -> (43.25, -32.0377)
  line L492 (43.25, -32.0377) -> (38.5, -34.7801)
  line L493 (-49.5, -23.8104) -> (-44.75, -26.5528)
  line L494 (-54.25, -26.5528) -> (-49.5, -23.8104)
  line L495 (-55, -25.2538) -> (-59.75, -22.5114)
  line L496 (-50.25, -22.5114) -> (-55, -25.2538)
  line L497 (-60.5, -23.8104) -> (-55.75, -26.5528)
  line L498 (-55.75, -26.5528) -> (-55.75, -32.0377)
  line L499 (-55.75, -32.0377) -> (-60.5, -34.7801)
  line L500 (-60.5, -34.7801) -> (-65.25, -32.0377)
  line L501 (-65.25, -32.0377) -> (-65.25, -26.5528)
  line L502 (-65.25, -26.5528) -> (-60.5, -23.8104)
  line L503 (-60.5, -23.8104) -> (-60.5, -34.7801) construction
  line L504 (-60.5, -29.2952) -> (-58.125, -25.1816) construction
  line L505 (-49.5, -34.7801) -> (-54.25, -32.0377)
  line L506 (-54.25, -32.0377) -> (-54.25, -26.5528)
  circle A4 centre (-16, -16.3271) radius 3.2
  circle A5 centre (-16, 15.6729) radius 3.2
  circle A6 centre (16, 15.6729) radius 3.2
  circle A7 centre (16, -16.3271) radius 3.2
  line L507 (-22, -20.3271) -> (22, -20.3271)
  point P0 (0, 0)
  point P1 (-33, -0.7164)
  point P2 (-30.625, 3.3972)
  point P3 (-22, -0.7164)
  point P4 (-19.625, 3.3972)
  point P5 (-11, -0.7164)
  point P6 (-8.625, 3.3972)
  point P7 (0, -0.7164)
  point P8 (2.375, 3.3972)
  point P9 (11, -0.7164)
  point P10 (13.375, 3.3972)
  point P11 (22, -0.7164)
  point P12 (24.375, 3.3972)
  point P13 (33, -0.7164)
  point P14 (35.375, 3.3972)
  point P15 (44, -0.7164)
  point P16 (46.375, 3.3972)
  point P17 (55, -0.7164)
  point P18 (57.375, 3.3972)
  point P19 (-44, -0.7164)
  point P20 (-14.125, 12.9235)
  point P21 (-5.5, 8.8099)
  point P22 (-3.125, 12.9235)
  point P23 (5.5, 9.5263)
  point P24 (-38.5, 8.8099)
  point P25 (-16.5, 8.8099)
  point P26 (5.5, 8.8099)
  point P27 (7.875, 12.9235)
  point P28 (16.5, 8.8099)
  point P29 (29.875, 12.9235)
  point P30 (38.5, 8.8099)
  point P31 (40.875, 12.9235)
  point P32 (27.5, 8.8099)
  point P33 (18.875, 12.9235)
  point P34 (-36.125, 12.9235)
  point P35 (-38.5, 8.8099)
  point P36 (-27.5, 8.8099)
  point P37 (-25.125, 12.9235)
  point P38 (49.5, 8.8099)
  point P39 (51.875, 12.9235)
  point P40 (60.5, 8.8099)
  point P41 (62.875, 12.9235)
  point P42 (-8.625, 22.4498)
  point P43 (0, 18.3362)
  point P44 (2.375, 22.4498)
  point P45 (11, 19.0526)
  point P46 (-33, 18.3362)
  point P47 (-11, 18.3362)
  point P48 (11, 18.3362)
  point P49 (13.375, 22.4498)
  point P50 (22, 18.3362)
  point P51 (35.375, 22.4498)
  point P52 (44, 18.3362)
  point P53 (46.375, 22.4498)
  point P54 (33, 18.3362)
  point P55 (24.375, 22.4498)
  point P56 (-30.625, 22.4498)
  point P57 (-33, 18.3362)
  point P58 (-22, 18.3362)
  point P59 (-19.625, 22.4498)
  point P60 (55, 18.3362)
  point P61 (57.375, 22.4498)
  point P62 (66, 18.3362)
  point P63 (68.375, 22.4498)
  point P64 (-3.125, 31.9761)
  point P65 (5.5, 27.8624)
  point P66 (7.875, 31.9761)
  point P67 (16.5, 28.5788)
  point P68 (-27.5, 27.8624)
  point P69 (-5.5, 27.8624)
  point P70 (16.5, 27.8624)
  point P71 (18.875, 31.9761)
  point P72 (27.5, 27.8624)
  point P73 (40.875, 31.9761)
  point P74 (49.5, 27.8624)
  point P75 (51.875, 31.9761)
  point P76 (38.5, 27.8624)
  point P77 (29.875, 31.9761)
  point P78 (-25.125, 31.9761)
  point P79 (-27.5, 27.8624)
  point P80 (-16.5, 27.8624)
  point P81 (-14.125, 31.9761)
  point P82 (60.5, 27.8624)
  point P83 (62.875, 31.9761)
  point P84 (71.5, 27.8624)
  point P85 (73.875, 31.9761)
  point P86 (27.5, -10.2427)
  point P87 (29.875, -6.1291)
  point P88 (16.5, -10.2427)
  point P89 (18.875, -6.1291)
  point P90 (-5.5, -9.5263)
  point P91 (5.5, -10.2427)
  point P92 (7.875, -6.1291)
  point P93 (-3.125, -6.1291)
  point P94 (-16.5, -10.2427)
  point P95 (-14.125, -6.1291)
  point P96 (-5.5, -10.2427)
  point P97 (-27.5, -10.2427)
  point P98 (-25.125, -6.1291)
  point P99 (38.5, -10.2427)
  point P100 (40.875, -6.1291)
  point P101 (49.5, -10.2427)
  point P102 (51.875, -6.1291)
  point P103 (-36.125, -6.1291)
  point P104 (-49.5, -10.2427)
  point P105 (-38.5, -10.2427)
  point P106 (22, -19.769)
  point P107 (24.375, -15.6553)
  point P108 (11, -19.769)
  point P109 (13.375, -15.6553)
  point P110 (-11, -19.0526)
  point P111 (0, -19.769)
  point P112 (2.375, -15.6553)
  point P113 (-8.625, -15.6553)
  point P114 (-22, -19.769)
  point P115 (-19.625, -15.6553)
  point P116 (-11, -19.769)
  point P117 (-33, -19.769)
  point P118 (-30.625, -15.6553)
  point P119 (33, -19.769)
  point P120 (35.375, -15.6553)
  point P121 (44, -19.769)
  point P122 (46.375, -15.6553)
  point P123 (-41.625, -15.6553)
  point P124 (-55, -19.769)
  point P125 (-44, -19.769)
  point P126 (16.5, -29.2952)
  point P127 (18.875, -25.1816)
  point P128 (5.5, -29.2952)
  point P129 (7.875, -25.1816)
  point P130 (-16.5, -28.5788)
  point P131 (-5.5, -29.2952)
  point P132 (-3.125, -25.1816)
  point P133 (-14.125, -25.1816)
  point P134 (-27.5, -29.2952)
  point P135 (-25.125, -25.1816)
  point P136 (-16.5, -29.2952)
  point P137 (-38.5, -29.2952)
  point P138 (-36.125, -25.1816)
  point P139 (27.5, -29.2952)
  point P140 (29.875, -25.1816)
  point P141 (38.5, -29.2952)
  point P142 (40.875, -25.1816)
  point P143 (-47.125, -25.1816)
  point P144 (-60.5, -29.2952)
  point P145 (-49.5, -29.2952)
  point P146 (17.25, -20.3271)
  point P147 (19.1735, -15.916)
  point P148 (17.25, -19.2729)
  point P149 (6.25, -20.3271)
  point P150 (15.75, -20.3271)
  point P151 (15.75, -19.5173)
  point P152 (12.9366, -15.4022)
  point P153 (-4.75, -20.3271)
  point P154 (4.75, -20.3271)
  point P155 (-12.9366, -15.4022)
  point P156 (-15.75, -19.5173)
  point P157 (-15.75, -20.3271)
  point P158 (-6.25, -20.3271)
  point P159 (-17.25, -20.3271)
  point P160 (-17.25, -19.2729)
  point P161 (-19.1735, -15.916)
  point P162 (-18.6268, -14.4996)
  point P163 (-13.6946, -14.1078)
  point P164 (13.6946, -14.1078)
  point P165 (18.6268, -14.4996)
  point P166 (-14.2485, 12.9948)
  point P167 (-18.1763, 13.3269)
  point P168 (-19.0073, 14.5792)
  point P169 (-17.25, 18.6187)
  point P170 (-17.25, 19.6729)
  point P171 (-6.25, 19.6729)
  point P172 (-15.75, 19.6729)
  point P173 (-15.75, 18.8631)
  point P174 (-13.2009, 14.122)
  point P175 (4.75, 19.6729)
  point P176 (-4.75, 19.6729)
  point P177 (13.2009, 14.122)
  point P178 (15.75, 18.8631)
  point P179 (15.75, 19.6729)
  point P180 (6.25, 19.6729)
  point P181 (18.1763, 13.3269)
  point P182 (14.2485, 12.9948)
  point P183 (19.0073, 14.5792)
  point P184 (17.25, 19.6729)
  point P185 (17.25, 18.6187)
  dimension "d30" = 9.5
  dimension "d31" = 3.4
  dimension "d34" = 32
  dimension "d37" = 32
  dimension "d42" = 11
  dimension "d47" = 22
  dimension "d50" = 11
  dimension "d57" = 11
  dimension "d62" = 1.5
  dimension "d63" = 1.5
  dimension "d64" = 1.5
  dimension "d65" = 1.5
  constraints: 1006 end point, 13 point on line, 8 centre point, 4 coincident, 4 horizontal, 3 collinear, 3 vertical, 2 midpoint, 1 parallel, 1175 other
  measures "d30" distance between parallel lines of L2 L5
  measures "d31" diameter of A0
  measures "d34" distance of L9.start L11.start
  measures "d37" distance of L9.start L15.start
  measures "d42" distance of L17.start point (-33, -0.716)
  measures "d47" distance from line of L10 point (-44, -0.716)
  measures "d50" distance of L24.end L72.start
  measures "d57" distance of L0.start L258.start
  measures "d62" radial gap between concentric circles of A4 A2
  measures "d63" radial gap between concentric circles of A5 A0
  measures "d64" radial gap between concentric circles of A6 A1
  measures "d65" radial gap between concentric circles of A3 A7
extrude "Extrusion5" cut sketch "Sketch5" against normal blind 10 contours A0 L144 L145 | L145 L144 A0 L74 L84 L179 L178 | L178 L179 A0 | L145 L14 L135 L134 L144 A5 | A0 L84 L74 | A5 L179 L10 L14 L178 | L74 L73 L72 L82 L83 L84 A5 | L14 L140 L139 L137 L143 | L26 L24 L25 L10 | L14 L155 A6 L150 L149 L147 | L371 A4 L376 L507 L10 | L14 L12 L153 A6 L152 | L371 L376 A2 | A2 L298 L297 L375 L377 L376 L371 | L298 L295 L291 L288 L293 L297 A4 | L155 L150 A1 | A1 L152 L153 L106 L92 L150 L155 | L377 A4 L375 L366 L358 L507 | A2 L297 L298 | A1 L153 L152 | A6 L106 L108 L107 L91 L90 L92 | L377 L375 A2 | L12 L51 L52 L53 | L92 L106 A1 | L363 L362 L361 L360 L507 | L12 L507 L346 A7 L347 | L355 L352 L353 A7 L354 L507 | L347 L346 A3 L354 L353 L273 L274 | A3 L346 L347 | A7 L273 L272 L269 L270 L271 L274 | L274 L273 A3 | A3 L353 L354 | L30 L31 L33 L34 L35 L32 | L36 L37 L39 L40 L41 L38 | L42 L43 L45 L46 L47 L44 | L75 L81 L76 L79 L78 L77 | L85 L86 L89 L93 L88 L87 | L275 L276 L296 L294 L292 L283 | L277 L282 L281 L280 L279 L278
body "Solid1"
